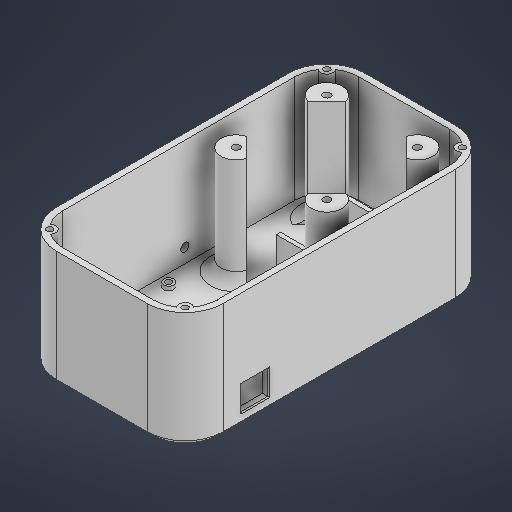
# Autodesk Inventor part: JoystickBox
Saved by Autodesk Inventor 2026.1 (Build 301233000, 233)
## iProperties
Created: 2026-01-14
Part Number: JoystickBox
Material: Generic
Document SubType Name: Modeling
Designer: Brynjar
Density: 1 g/cm^3
Appearance: Default
Author: Brynjar
Autodesk Inventor part; units mm, degrees
ref_plane "YZ Plane" through (0, 0, 0) normal (1, 0, 0) x (0, 1, 0)
ref_plane "XZ Plane" through (0, 0, 0) normal (0, 1, 0) x (-1, 0, 0)
ref_plane "XY Plane" through (0, 0, 0) normal (0, 0, 1) x (1, 0, 0)
sketch "Sketch1" plane through (0, 0, 0) normal (0, 1, 0) x (-1, 0, 0)
  line L0 (22, 22) -> (-22, 22) construction
  line L1 (-22, 22) -> (-22, -22) construction
  line L2 (-22, -22) -> (22, -22) construction
  line L3 (22, -22) -> (22, 22) construction
  line L4 (22, 22) -> (-22, -22) construction
  line L5 (-22, 22) -> (22, -22) construction
  circle A0 centre (22, -22) radius 1.8
  circle A1 centre (-22, -22) radius 1.8
  circle A2 centre (-22, 22) radius 1.8
  circle A3 centre (22, 22) radius 1.8
  line L6 (25, -11) -> (25, 11) construction
  line L7 (-25, -11) -> (-25, 11) construction
  line L8 (-25, 11) -> (-11, 25) construction
  line L9 (-11, 25) -> (11, 25) construction
  line L10 (11, 25) -> (25, 11) construction
  line L11 (25, -11) -> (11, -25) construction
  line L12 (11, -25) -> (-11, -25) construction
  line L13 (-11, -25) -> (-25, -11) construction
  line L14 (25, 0) -> (-25, 0) construction
  line L15 (0, 25) -> (0, -25) construction
  line L16 (-11.8284, -27) -> (11.8284, -27)
  line L17 (11.8284, -27) -> (27, -11.8284)
  line L18 (27, -11.8284) -> (27, 11.8284)
  line L19 (27, 11.8284) -> (11.8284, 27)
  line L20 (11.8284, 27) -> (-11.8284, 27)
  line L21 (-11.8284, 27) -> (-27, 11.8284)
  line L22 (-27, 11.8284) -> (-27, -11.8284)
  line L23 (-27, -11.8284) -> (-11.8284, -27)
  circle A4 centre (22, -22) radius 7.5
  circle A5 centre (-22, -22) radius 7.5
  circle A6 centre (-22, 22) radius 7.5
  circle A7 centre (22, 22) radius 7.5
  point P0 (0, 0)
  point P1 (24.0444, 14.784)
  point P2 (14.784, 24.0444)
  point P3 (-14.784, 24.0444)
  point P4 (-24.0444, 14.784)
  point P5 (14.784, -24.0444)
  point P6 (24.0444, -14.784)
  point P7 (-24.0444, -14.784)
  point P8 (-14.784, -24.0444)
  dimension "d1" = 44
  dimension "d2" = 3.6
  dimension "d4" = 50
  dimension "d5" = 22
  dimension "d6" = 2
  dimension "d65" = 15
  constraints: 48 end point, 8 centre point, 8 coincident, 8 midpoint, 8 parallel, 6 equal radius, 5 perpendicular, 4 equal length, 3 vertical, 2 horizontal, 7 other
  measures "d1" distance of L1.end L0.end
  measures "d2" diameter of A3
  measures "d4" distance between parallel lines of L9 L12
  measures "d5" distance of L8.end L9.end
  measures "d6" distance between parallel lines of L12 L16
  measures "d65" diameter of A7
extrude "Extrusion1" add sketch "Sketch1" against normal blind 32 contours A5 L23 | L17 A4 | A6 L21 | L19 A7 picked at (-19.827, -19.8783) picked at (19.827, -19.8783) picked at (-19.827, 19.8783) picked at (19.827, 19.8783)
sketch "Sketch2" plane through (0, -32, 0) normal (0, -1, 0) x (1, 0, 0)
  line L0 (14.784, 24.0444) -> (24.0444, 14.784) projected
  arc A0 (24.0444, 14.784) -> (14.784, 24.0444) centre (22, 22) ccw projected
  circle A1 centre (22, 22) radius 1.8 projected
  line L1 (24.0444, -14.784) -> (14.784, -24.0444) projected
  arc A2 (14.784, -24.0444) -> (24.0444, -14.784) centre (22, -22) ccw projected
  circle A3 centre (22, -22) radius 1.8 projected
  line L2 (-14.784, -24.0444) -> (-24.0444, -14.784) projected
  arc A4 (-24.0444, -14.784) -> (-14.784, -24.0444) centre (-22, -22) ccw projected
  circle A5 centre (-22, -22) radius 1.8 projected
  line L3 (-24.0444, 14.784) -> (-14.784, 24.0444) projected
  arc A6 (-14.784, 24.0444) -> (-24.0444, 14.784) centre (-22, 22) ccw projected
  circle A7 centre (-22, 22) radius 1.8 projected
  line L4 (0, 15) -> (0, -15) construction
  line L5 (7.5, -15) -> (-7.5, -15)
  line L6 (-7.5, -15) -> (-7.5, -17)
  line L7 (-7.5, -17) -> (7.5, -17)
  line L8 (7.5, -17) -> (7.5, -15)
  line L9 (7.5, 17) -> (-7.5, 17)
  line L10 (-7.5, 17) -> (-7.5, 15)
  line L11 (-7.5, 15) -> (7.5, 15)
  line L12 (7.5, 15) -> (7.5, 17)
  line L13 (17, 7.5) -> (15, 7.5)
  line L14 (15, 7.5) -> (15, -7.5)
  line L15 (15, -7.5) -> (17, -7.5)
  line L16 (17, -7.5) -> (17, 7.5)
  line L17 (-15, 0) -> (15, 0) construction
  point P0 (0, 0)
  point P1 (0, 0)
  dimension "d9" = 30
  dimension "d10" = 2
  dimension "d11" = 15
  constraints: 28 end point, 8 perpendicular, 6 parallel, 5 midpoint, 4 horizontal, 1 coincident, 1 vertical
  measures "d9" distance of L4.start L4.end
  measures "d10" distance of L14.end L15.end
  measures "d11" distance of L15.end L13.start
extrude "Extrusion2" add sketch "Sketch2" along normal blind 20
sketch "Sketch3" plane through (0, -52, 0) normal (0, -1, 0) x (1, 0, 0)
  line L0 (37.5, 90.9) -> (37.5, -22)
  line L1 (22, -37.5) -> (-22, -37.5)
  line L2 (-37.5, -22) -> (-37.5, 90.9)
  arc A0 (22, -37.5) -> (37.5, -22) centre (22, -22) ccw
  arc A1 (-37.5, -22) -> (-22, -37.5) centre (-22, -22) ccw
  circle A2 centre (22, -22) radius 1.8 construction
  circle A3 centre (-22, -22) radius 1.8 construction
  line L3 (-34.3, 90.9) -> (34.3, 90.9) construction
  line L4 (34.3, 90.9) -> (34.3, 37.5) construction
  line L5 (34.3, 37.5) -> (-34.3, 37.5) construction
  line L6 (-34.3, 37.5) -> (-34.3, 90.9) construction
  line L7 (0, 90.9) -> (0, 37.5) construction
  line L8 (22, 106.4) -> (-22, 106.4)
  arc A4 (37.5, 90.9) -> (22, 106.4) centre (22, 90.9) ccw
  arc A5 (-22, 106.4) -> (-37.5, 90.9) centre (-22, 90.9) ccw
  line L9 (0, 37.5) -> (0, 17) construction
  line L10 (7.5, 17) -> (-7.5, 17) construction
  line L11 (-7.5, -17) -> (7.5, -17) construction
  line L12 (0, -17) -> (0, -37.5) construction
  circle A6 centre (-31.8, 73) radius 1.5
  circle A7 centre (-31.8, 45.1) radius 1.5
  circle A8 centre (19, 88.2) radius 1.5
  circle A9 centre (20.3, 40) radius 1.5
  line L13 (-31.8, 73) -> (-31.8, 45.1) construction
  line L14 (-40.5, 90.9) -> (-40.5, -22)
  arc A10 (-40.5, -22) -> (-22, -40.5) centre (-22, -22) ccw
  line L15 (-22, -40.5) -> (22, -40.5)
  arc A11 (22, -40.5) -> (40.5, -22) centre (22, -22) ccw
  line L16 (40.5, -22) -> (40.5, 90.9)
  arc A12 (40.5, 90.9) -> (22, 109.4) centre (22, 90.9) ccw
  line L17 (22, 109.4) -> (-22, 109.4)
  arc A13 (-22, 109.4) -> (-40.5, 90.9) centre (-22, 90.9) ccw
  line L18 (40.5, 81.3) -> (23.5, 81.3) construction
  line L19 (23.5, 81.3) -> (23.5, 69.3) construction
  line L20 (23.5, 69.3) -> (40.5, 69.3) construction
  line L21 (40.5, 69.3) -> (40.5, 81.3) construction
  circle A14 centre (19, 88.2) radius 2.5
  circle A15 centre (20.3, 40) radius 2.5
  circle A16 centre (-31.8, 73) radius 2.5
  circle A17 centre (-31.8, 45.1) radius 2.5
  point P0 (0, 0)
  dimension "d17" = 75
  dimension "d18" = 68.6
  dimension "d19" = 53.4
  dimension "d26" = 27.9
  dimension "d28" = 1.3
  dimension "d29" = 15.2
  dimension "d30" = 5.1
  dimension "d31" = 3
  dimension "d32" = 2.5
  dimension "d33" = 14
  dimension "d34" = 50.8
  dimension "d35" = 3
  dimension "d40" = 6.2
  dimension "d41" = 9.6
  dimension "d42" = 12
  dimension "d43" = 17
  dimension "d44" = 5
  constraints: 40 end point, 16 centre point, 16 point on circle, 8 tangent, 7 equal radius, 6 coincident, 6 parallel, 5 midpoint, 4 horizontal, 3 vertical, 2 equal length, 2 perpendicular, 2 point on line, 7 other
  measures "d17" distance between parallel lines of L2 L0
  measures "d18" distance of L4.end L5.end
  measures "d19" distance of L3.end L4.end
  measures "d26" distance of L13.end L13.start
  measures "d28" horizontal distance of A8.centre A9.centre
  measures "d29" vertical distance of L13.start A8.centre
  measures "d30" vertical distance of A9.centre L13.end
  measures "d31" diameter of A6
  measures "d32" distance from line of L5 A9.centre
  measures "d33" distance from line of L4 A9.centre
  measures "d34" horizontal distance of L13.start A8.centre
  measures "d35" distance between parallel lines of L2 L14
  measures "d40" distance between parallel lines of L4 L21
  measures "d41" distance between parallel lines of L3 L18
  measures "d42" distance of L20.end L18.start
  measures "d43" distance of L19.end L20.end
  measures "d44" diameter of A16
extrude "Extrusion3" add sketch "Sketch3" along normal blind 5 contours L0 A0 L1 A1 L2 A5 L8 A4 | A13 L17 A12 L16 A11 L15 A10 L14 | A14 | A15 | A16 | A17
sketch "Sketch4" plane through (0, -52, 0) normal (0, 1, 0) x (1, 0, 0)
  arc A0 (-22, 40.5) -> (-40.5, 22) centre (-22, 22) ccw projected
  line L0 (-40.5, -90.9) -> (-40.5, 22) projected
  arc A1 (-40.5, -90.9) -> (-22, -109.4) centre (-22, -90.9) ccw projected
  line L1 (22, -109.4) -> (-22, -109.4) projected
  arc A2 (22, -109.4) -> (40.5, -90.9) centre (22, -90.9) ccw projected
  line L2 (40.5, 22) -> (40.5, -90.9) projected
  arc A3 (40.5, 22) -> (22, 40.5) centre (22, 22) ccw projected
  line L3 (-22, 40.5) -> (22, 40.5) projected
  circle A4 centre (20.3, -40) radius 1.5 projected
  circle A5 centre (19, -88.2) radius 1.5 projected
  circle A6 centre (-31.8, -45.1) radius 1.5 projected
  circle A7 centre (-31.8, -73) radius 1.5 projected
  line L4 (7.5, -17) -> (-7.5, -17) projected
  line L5 (-7.5, -17) -> (-7.5, -15) projected
  line L6 (-7.5, -15) -> (7.5, -15) projected
  line L7 (7.5, -15) -> (7.5, -17) projected
  line L8 (7.5, 15) -> (-7.5, 15) projected
  line L9 (-7.5, 15) -> (-7.5, 17) projected
  line L10 (-7.5, 17) -> (7.5, 17) projected
  line L11 (7.5, 17) -> (7.5, 15) projected
  line L12 (17, -7.5) -> (15, -7.5) projected
  line L13 (15, -7.5) -> (15, 7.5) projected
  line L14 (15, 7.5) -> (17, 7.5) projected
  line L15 (17, 7.5) -> (17, -7.5) projected
  arc A8 (14.784, -24.0444) -> (24.0444, -14.784) centre (22, -22) ccw projected
  line L16 (14.784, -24.0444) -> (24.0444, -14.784) projected
  arc A9 (-14.784, 24.0444) -> (-24.0444, 14.784) centre (-22, 22) ccw projected
  line L17 (-14.784, 24.0444) -> (-24.0444, 14.784) projected
  arc A10 (-24.0444, -14.784) -> (-14.784, -24.0444) centre (-22, -22) ccw projected
  line L18 (-24.0444, -14.784) -> (-14.784, -24.0444) projected
  arc A11 (24.0444, 14.784) -> (14.784, 24.0444) centre (22, 22) ccw projected
  line L19 (24.0444, 14.784) -> (14.784, 24.0444) projected
  arc A12 (-22, 37.5) -> (-37.5, 22) centre (-22, 22) ccw
  line L20 (-22, 37.5) -> (22, 37.5)
  arc A13 (37.5, 22) -> (22, 37.5) centre (22, 22) ccw
  line L21 (37.5, 22) -> (37.5, -90.9)
  arc A14 (22, -106.4) -> (37.5, -90.9) centre (22, -90.9) ccw
  line L22 (22, -106.4) -> (-22, -106.4)
  arc A15 (-37.5, -90.9) -> (-22, -106.4) centre (-22, -90.9) ccw
  line L23 (-37.5, -90.9) -> (-37.5, 22)
  point P0 (22, -88.4)
  dimension "d36" = 3
  constraints: 8 end point, 8 point on circle, 4 centre point, 7 other
  measures "d36" distance between parallel lines of L0 L23
extrude "Extrusion4" add sketch "Sketch4" along normal up to surface (52 mm away) contours L3 A3 L2 A2 L1 A1 L0 A0
sketch "Sketch5" plane through (-40.5, -57, -22) normal (-1, 0, 0) x (0, 0, 1)
  line L0 (0, 5) -> (112.9, 5) construction
  line L1 (51.5, 57) -> (51.5, 5) construction
  circle A0 centre (53.5, 12) radius 2
  line L2 (51.5, 10) -> (53.5, 10) construction
  point P0 (22, 57)
  dimension "d37" = 4
  dimension "d54" = 5
  constraints: 2 end point, 1 horizontal, 1 point on line, 1 vertical, 1 vertical alignment, 2 other
  measures "d54" distance between parallel lines of L0 L2
extrude "Extrusion5" cut sketch "Sketch5" against normal up to next
extrude "Extrusion6" add sketch "Sketch3" against normal blind 2 contours A14 | A15 | A16 | A17
sketch "Sketch6" plane through (40.5, -57, 90.9) normal (1, 0, 0) x (0, 0, -1)
  line L0 (1.2, 7) -> (4.2, 7) construction
  line L1 (49.4, 7) -> (52.4, 7) construction
  line L2 (9.6, 5) -> (21.6, 5) construction
  line L3 (9.1, 6.6) -> (22.1, 6.6)
  line L4 (9.1, 6.6) -> (9.1, 18.5)
  line L5 (9.1, 18.5) -> (22.1, 18.5)
  line L6 (22.1, 18.5) -> (22.1, 6.6)
  line L7 (15.6, 5) -> (15.6, 6.6) construction
  point P0 (90.9, 57)
  dimension "d47" = 1.6
  dimension "d48" = 13
  dimension "d49" = 11.9
  constraints: 10 end point, 2 midpoint, 2 perpendicular, 2 vertical, 1 horizontal
  measures "d47" distance between parallel lines of L3 L2
  measures "d48" distance of L4.end L5.end
  measures "d49" distance of L5.end L3.end
extrude "Extrusion7" cut sketch "Sketch6" against normal up to next
fillet "Fillet1" radius 0.5 4 edges at (40.5, -38.5, 75.3) (40.5, -44.45, 68.8) (40.5, -50.4, 75.3) (40.5, -44.45, 81.8)
sketch "Sketch7" plane through (-22, 0, -40.5) normal (0, 1, 0) x (1, 0, 0)
  circle A0 centre (-10.9602, -7.5398) radius 1.5
  arc A1 (0, -3) -> (-15.5, -18.5) centre (0, -18.5) ccw construction
  circle A2 centre (-10.9602, -7.5398) radius 3
  arc A3 (0, 0) -> (-18.5, -18.5) centre (0, -18.5) ccw construction
  arc A4 (-18.5, -131.4) -> (0, -149.9) centre (0, -131.4) ccw construction
  arc A5 (-15.5, -131.4) -> (0, -146.9) centre (0, -131.4) ccw construction
  arc A6 (44, -149.9) -> (62.5, -131.4) centre (44, -131.4) ccw construction
  arc A7 (44, -146.9) -> (59.5, -131.4) centre (44, -131.4) ccw construction
  arc A8 (59.5, -18.5) -> (44, -3) centre (44, -18.5) ccw construction
  arc A9 (62.5, -18.5) -> (44, 0) centre (44, -18.5) ccw construction
  circle A10 centre (-10.9602, -142.3602) radius 1.5
  circle A11 centre (54.9602, -142.3602) radius 1.5
  circle A12 centre (54.9602, -7.5398) radius 1.5
  circle A13 centre (-10.9602, -142.3602) radius 3
  circle A14 centre (54.9602, -142.3602) radius 3
  circle A15 centre (54.9602, -7.5398) radius 3
  point P0 (22, -40.5)
  dimension "d55" = 3
  constraints: 8 centre point, 4 coincident, 4 point on circle, 4 tangent, 3 equal radius
  measures "d55" diameter of A0
extrude "Extrusion8" cut sketch "Sketch7" against normal up to surface (52 mm away) contours A0 | A10 | A11 | A12
extrude "Extrusion9" add sketch "Sketch7" against normal up to surface (52 mm away)
chamfer "Chamfer1" distance 3 angle 45 8 edges at (40.5, -57, 34.45) (35.0815, -57, 103.9815) (0, -57, 109.4) (-35.0815, -57, 103.9815) (-40.5, -57, 34.45) (-35.0815, -57, -35.0815) (0, -57, -40.5) (35.0815, -57, -35.0815)
fillet "Fillet3" radius 5 4 edges at (-27.3033, -52, 27.3033) (27.3033, -52, 27.3033) (-27.3033, -52, -27.3033) (27.3033, -52, -27.3033)
body "Solid1"
